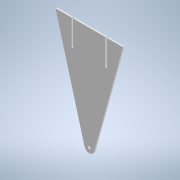
# Autodesk Inventor part: Pivote_Estructura
Saved by Autodesk Inventor 2022 (Build 260153000, 153)
## iProperties
Created: 2022-01-30
Part Number: Pivote_Estructura
Material: Generic
Document SubType Name: Modeling
Designer: katha
Density: 1 g/cm^3
Appearance: Default
Author: katha
Autodesk Inventor part; units mm, degrees
ref_plane "YZ Plane" through (0, 0, 0) normal (1, 0, 0) x (0, 1, 0)
ref_plane "XZ Plane" through (0, 0, 0) normal (0, 1, 0) x (-1, 0, 0)
ref_plane "XY Plane" through (0, 0, 0) normal (0, 0, 1) x (1, 0, 0)
sketch "Sketch1" plane through (0, 0, 0) normal (0, 0, 1) x (1, 0, 0)
  circle A0 centre (0, 16.5) radius 2.5 projected
  line L0 (0, 16.5) -> (0, 216.5) construction
  arc A1 (-9.1582, 13.9748) -> (9.1582, 13.9748) centre (0, 16.5) ccw
  line L1 (65, 216.5) -> (9.1582, 13.9748)
  circle A2 centre (0, 16.5) radius 2.5
  line L2 (34, 216.5) -> (34, 166.5)
  line L3 (34, 166.5) -> (31, 166.5)
  line L4 (31, 166.5) -> (31, 216.5)
  line L5 (0, 216.5) -> (31, 216.5)
  line L6 (34, 216.5) -> (65, 216.5)
  line L7 (-65, 216.5) -> (-9.1582, 13.9748)
  line L8 (-34, 216.5) -> (-34, 166.5)
  line L9 (-34, 166.5) -> (-31, 166.5)
  line L10 (-31, 166.5) -> (-31, 216.5)
  line L11 (0, 216.5) -> (-31, 216.5)
  line L12 (-34, 216.5) -> (-65, 216.5)
  point P0 (0, 0)
  dimension "d0" = 200
  dimension "d1" = 65
  dimension "d2" = 19
  dimension "d7" = 50
  dimension "d8" = 3
  dimension "d9" = 31
  constraints: 26 end point, 6 symmetric about line, 3 perpendicular, 2 centre point, 2 coincident, 2 horizontal, 2 point on circle, 2 vertical, 1 concentric, 1 parallel, 1 tangent
  measures "d0" distance of L0.start L0.end
  measures "d1" distance of L0.end L1.start
  measures "d2" diameter of A1
  measures "d7" distance of L2.start L2.end
  measures "d8" distance of L2.end L3.end
  measures "d9" distance of L2.start L1.start
extrude "Extrusion2" add sketch "Sketch1" along normal blind 1.5 and the other way blind 1.5
body "Solid2"
